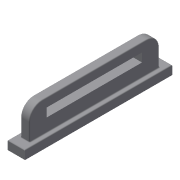
# Autodesk Inventor part: Part5
Saved by Autodesk Inventor 2014 (Build 180170000, 170)
## iProperties
Created: 2013-07-16
Part Number: Part5
Material: Generic
Document SubType Name: Modeling
Density: 1 g/cm^3
Appearance: Default
Autodesk Inventor part; units mm, degrees
ref_plane "YZ Plane" through (0, 0, 0) normal (1, 0, 0) x (0, 1, 0)
ref_plane "XZ Plane" through (0, 0, 0) normal (0, 1, 0) x (-1, 0, 0)
ref_plane "XY Plane" through (0, 0, 0) normal (0, 0, 1) x (1, 0, 0)
sketch "Sketch1" plane through (0, 0, 0) normal (1, 0, 0) x (0, 1, 0)
  line L0 (-150, 0) -> (150, 0)
  line L1 (150, 0) -> (150, 40)
  line L2 (120, 70) -> (-120, 70)
  line L3 (-150, 40) -> (-150, 0)
  line L4 (0, 0) -> (0, 116.1684) construction
  arc A0 (-120, 70) -> (-150, 40) centre (-120, 40) ccw
  arc A1 (150, 40) -> (120, 70) centre (120, 40) ccw
  line L5 (-110, 50) -> (110, 50)
  line L6 (110, 50) -> (110, 30)
  line L7 (110, 30) -> (-110, 30)
  line L8 (-110, 30) -> (-110, 50)
  point P0 (-150, 70)
  dimension "d0" = 300
  dimension "d1" = 70
  dimension "d2" = 30
  dimension "d3" = 220
  dimension "d4" = 20
  dimension "d5" = 30
  constraints: 18 end point, 5 parallel, 4 point on circle, 4 tangent, 2 centre point, 2 horizontal, 2 perpendicular, 2 point on line, 1 equal radius, 1 vertical, 2 other
  measures "d0" distance of L0.start L0.end
  measures "d1" distance of point (-150, 70) L0.start
  measures "d2" radius of A0
  measures "d3" distance between parallel lines of L6 L8
  measures "d4" distance of L7.end L5.start
  measures "d5" distance between parallel lines of L0 L7
extrude "Extrusion1" add sketch "Sketch1" along normal mid plane 20
sketch "Sketch2" plane through (0, 0, 0) normal (1, 0, 0) x (0, 1, 0)
  line L0 (-170, 0) -> (170, 0)
  line L1 (170, 0) -> (170, -20)
  line L2 (170, -20) -> (-170, -20)
  line L3 (-170, -20) -> (-170, 0)
  line L4 (0, 0) -> (0, 104.8066) construction
  line L5 (150, 0) -> (-150, 0) construction
  dimension "d8" = 340
  dimension "d9" = 20
  constraints: 10 end point, 3 parallel, 1 collinear, 1 horizontal, 1 perpendicular, 1 vertical, 1 other
  measures "d8" distance of L1.end L2.end
  measures "d9" distance of L2.end L0.start
extrude "Extrusion2" add sketch "Sketch2" along normal mid plane 40
fillet "Fillet1" radius 2 18 edges at (0, -170, 0) (20, 0, 0) (0, 170, 0) (-20, 0, 0) (10, 0, 0) (10, 150, 20) (10, 141.2132, 61.2132) (10, 0, 70) (10, -141.2132, 61.2132) (10, -150, 20) (-10, -141.2132, 61.2132) (-10, 0, 70) (-10, 141.2132, 61.2132) (-10, 150, 20) (-10, -150, 20) (-10, 0, 0) (0, -150, 0) (0, 150, 0)
body "Solid1"
